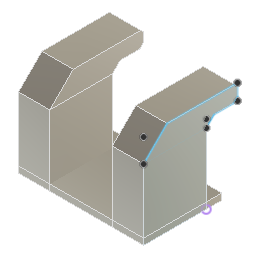
держатель киянки или молотка (Autodesk Fusion 360 design; units mm, degrees)
Autodesk Fusion 360 part; units mm, degrees
note: some values were not read from the file. Chosen so that the rebuilt part matches the saved one: which face or edge a step refers to. Set by a fixed rule: which sketch regions a step uses.
sketch "Sketch1" plane through (0, 0, 0) normal (0, 0, 1) x (1, 0, 0)
  line L0 (20, 20) -> (-20, 20)
  line L1 (-20, 20) -> (-20, -20)
  line L2 (-20, -20) -> (20, -20)
  line L3 (20, -20) -> (20, 20)
  line L4 (40, 20) -> (-40, 20)
  line L5 (-40, 20) -> (-40, -20)
  line L6 (-40, -20) -> (40, -20)
  line L7 (40, -20) -> (40, 20)
  circle A0 centre (-10, 15) radius 2
  circle A1 centre (10, 15) radius 2
  line L8 (-40, 20) -> (-40, 30)
  line L9 (-40, 30) -> (40, 30)
  line L10 (40, 30) -> (40, 20)
  constraint horizontal L0
  constraint perpendicular L0 L1
  constraint parallel L0 L2
  constraint parallel L1 L3
  constraint horizontal L4
  constraint perpendicular L4 L5
  constraint parallel L4 L6
  constraint parallel L5 L7
  constraint perpendicular L4 L8
  constraint perpendicular L8 L9
  constraint perpendicular L4 L10
extrude "Extrude1" add sketch "Sketch1" along normal blind 4 makes body 1
extrude "Extrude2" add sketch "Sketch1" along normal blind 45 contours L3 L4 L6 L7 | L1 L4 L5 L6 makes body 2 at (-20, 6.6667, 30) makes body 3 at (40, -6.6667, 30)
sketch "Sketch4" plane through (40, 0, 0) normal (1, 0, 0) x (0, 1, 0)
  line L0 (-20, 0) -> (20, 0)
  line L1 (20, 0) -> (20, 45)
  line L2 (20, 45) -> (-20, 45)
  line L3 (-20, 45) -> (-20, 0)
  line L4 (20, 45) -> (20, 45)
  line L5 (25, 50) -> (37.5, 50)
  line L6 (40, 52.5) -> (40, 58.125)
  line L7 (38.125, 60) -> (-5, 60)
  line L8 (-20, 45) -> (-20, 45)
  line L9 (20, 45) -> (25, 50)
  line L10 (-5, 60) -> (-20, 45)
  line L11 (37.5, 50) -> (40, 52.5)
  line L12 (40, 58.125) -> (38.125, 60)
  point P0 (20, 50)
  point P1 (40, 50)
  point P2 (40, 60)
  point P3 (-20, 60)
  dimension "d5" = 5
  dimension "d6" = 5
  dimension "d7" = 15
  dimension "d8" = 15
  dimension "d9" = 2.5
  dimension "d10" = 2.5
  dimension "d11" = 1.875
  dimension "d12" = 1.875
  constraint coincident L1.end L2.start
  constraint perpendicular L1 L5
  constraint perpendicular L5 L6
  constraint perpendicular L6 L7
  constraint coincident L2.end L3.start
  constraint coincident P0 L4
  constraint coincident P0 L5
  constraint coincident P3 L7
  constraint coincident P3 L8
  constraint coincident P1 L5
  constraint coincident P1 L6
  constraint coincident P2 L6
  constraint coincident P2 L7
  measures "d5" distance of P0 L1.end
  measures "d6" distance of P0 L5.start
  measures "d7" distance of P3 L7.end
  measures "d8" distance of P3 L2.end
  measures "d9" distance of P1 L5.end
  measures "d10" distance of P1 L6.start
  measures "d11" distance of P2 L6.end
  measures "d12" distance of P2 L7.start
extrude "Extrude3" add sketch "Sketch4" against normal blind 20 contours L2 L5 L6 L7 L9 L10 L11 L12 bodies 3
extrude "Extrude4" add sketch "Sketch4" along normal blind -80 and the other way blind 60 contours L2 L5 L6 L7 L9 L10 L11 L12 bodies 3 makes body 4
chamfer "Chamfer1" distance 1 angle 45 2 edges at (8, 15, 4) (-12, 15, 4) on bodies 1
chamfer "Chamfer2" [no effect]
equation "d6 = d5"
equation "d8 = d7"
equation "d10 = d9"
equation "d12 = d11"
